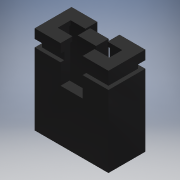
# Autodesk Inventor part: SNT-100-BK_body
Saved by Autodesk Inventor 2019 (Build 230136000, 136)
## iProperties
Category: PARTsolutions
Company: SAMTEC
Created: 2019-03-13
Part Number: SNT-100-BK_body
Material: Generico
Catalog Web Link: www.cadenas.de
Description: SNT Body-SNT Series - (2,54 mm) .100" Shunt
Vendor: SAMTEC
Document SubType Name: Modeling
Designer: psadmin
Manufacturer: SAMTEC
Mass: 0.0460404 g
Surface Area: 1.85169 cm^2
Volume: 0.0460404 cm^3
Density: 1 g/cm^3
Appearance: PSOLRGB-127-127-127
PSOL_IDENT_0: {$CADENAS_DATA\23d-libs\samtec\modelling\snt\parts\snt_body.prj},182 {VTYP=3D},{NB=SNT-100-BK_body},
PSOL_IDENT_1: {LINA=SNT-100-BK_body},{NN=SNT Body},{DATE=22.01.2016 08:16:46},{GEOMDATE=19.01.2016 13:08:00},{VERS
PSOL_IDENT_2: ION=},{LINEID=10},{WBVAR=COLOR,HOPT},{WBNUMERIC=}  {NB=SNT-100-BK_body},{LINA=SNT-100-BK_body},{KT=D
PSOL_IDENT_3: UMMY},{PN=SNT-100-BK},{SERIES=SNT},{COLOR=BK},{HOPTALG=   ''  , 'Not Selected' , 'H' , 'Handle'  },{
PSOL_IDENT_4: HOPT=},{A=0.240},{W=0.100},{L=0.200},{PINW=0.040},{HPN=},{COL=0.50,0.50,0.50,0.00}
NN: SNT Body
NT: SNT Series - (2,54 mm) .100" Shunt
NB: SNT-100-BK_body
NBSYN: $PN._body
LINA: SNT-100-BK_body
PN: SNT-100-BK
SERIES: SNT
COLOR: Black
HOPT: Not Selected
A: 0.24
W: 0.1
L: 0.2
PINW: 0.04
SUPPLIER: SAMTEC
ARTICLENO: SNT-100-BK_body
BOMINFO: SNT-100-BK_body
CREATOR: CADENAS GmbH
Title: SNT-100-BK_body
Author: Cadenas PARTsolutions
Comments: SNT Series - (2,54 mm) .100" Shunt
Autodesk Inventor part; units mm, degrees
sketch "Sketch_1" plane through (0, 0, 0) normal (0, 1, 0) x (1, 0, 0)
  line L0 (-2.54, 1.27) -> (-2.54, -1.27)
  line L1 (-2.54, -1.27) -> (2.54, -1.27)
  line L2 (2.54, -1.27) -> (2.54, 1.27)
  line L3 (2.54, 1.27) -> (-2.54, 1.27)
  constraints: 8 end point
extrude "Extrusion1" add sketch "Sketch_1" along normal blind 6.096
sketch "Sketch_2" plane through (0, 5.461, 0) normal (0, 1, 0) x (1, 0, 0)
  line L0 (-2.794, 2.54) -> (-2.794, -2.54)
  line L1 (-2.794, -2.54) -> (2.794, -2.54)
  line L2 (2.794, -2.54) -> (2.794, 2.54)
  line L3 (2.794, 2.54) -> (-2.794, 2.54)
  line L4 (-2.286, 1.016) -> (-2.286, -1.016)
  line L5 (-2.286, -1.016) -> (2.286, -1.016)
  line L6 (2.286, -1.016) -> (2.286, 1.016)
  line L7 (2.286, 1.016) -> (-2.286, 1.016)
  constraints: 16 end point
extrude "Extrusion2" cut sketch "Sketch_2" against normal blind 0.508
sketch "Sketch_3" plane through (0, 6.096, 0) normal (0, 1, 0) x (1, 0, 0)
  line L0 (-0.762, 1.27) -> (-0.762, -1.27)
  line L1 (-0.762, -1.27) -> (0.762, -1.27)
  line L2 (0.762, -1.27) -> (0.762, 1.27)
  line L3 (0.762, 1.27) -> (-0.762, 1.27)
  constraints: 8 end point
extrude "Extrusion3" cut sketch "Sketch_3" against normal blind 2.54
sketch "Sketch_4" plane through (0, 6.096, 0) normal (0, 1, 0) x (1, 0, 0)
  line L0 (-1.778, 0.4445) -> (-1.778, -0.4445)
  line L1 (-1.778, -0.4445) -> (1.778, -0.4445)
  line L2 (1.778, -0.4445) -> (1.778, 0.4445)
  line L3 (1.778, 0.4445) -> (-1.778, 0.4445)
  constraints: 8 end point
extrude "Extrusion4" cut sketch "Sketch_4" against normal blind 6.096
sketch "Sketch_5" plane through (0, 5.7912, 0) normal (0, 1, 0) x (1, 0, 0)
  line L0 (-2.032, 0.5969) -> (-2.032, -0.5969)
  line L1 (-2.032, -0.5969) -> (2.032, -0.5969)
  line L2 (2.032, -0.5969) -> (2.032, 0.5969)
  line L3 (2.032, 0.5969) -> (-2.032, 0.5969)
  constraints: 8 end point
extrude "Extrusion5" cut sketch "Sketch_5" against normal blind 6.096
sketch "Sketch_8" plane through (0, 0, 0) normal (0, 1, 0) x (-1, 0, 0)
  line L0 (0.762, -0.6477) -> (0.762, 0.6477)
  line L1 (0.762, 0.6477) -> (-0.762, 0.6477)
  line L2 (-0.762, 0.6477) -> (-0.762, -0.6477)
  line L3 (-0.762, -0.6477) -> (0.762, -0.6477)
  constraints: 8 end point
extrude "Extrusion6" cut sketch "Sketch_8" along normal blind 3.556
sketch "Sketch_6" plane through (0, 0, 0) normal (1, 0, 0) x (0, 1, 0)
  line L0 (3.0093, 0.2159) -> (2.2752, -0.6477)
  line L1 (2.2752, -0.6477) -> (6.096, -0.6477)
  line L2 (6.096, -0.6477) -> (6.096, 0.2159)
  line L3 (6.096, 0.2159) -> (3.0093, 0.2159)
  constraints: 8 end point
extrude "Extrusion7" add sketch "Sketch_6" along normal mid plane 1.27
ref_plane "body_to_dummy_XY" through (0, 0, 0) normal (0, -1, 0) x (1, 0, 0)
ref_plane "body_to_dummy_YZ" through (0, 0, 0) normal (1, 0, 0) x (0, 0, 1)
ref_plane "body_to_dummy_ZX" through (0, 0, 0) normal (0, 0, 1) x (0, -1, 0)
body "Solid1"
